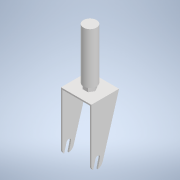
# Autodesk Inventor part: frontwheelFork
Saved by Autodesk Inventor 2022.2 (Build 262287010, 287A)
## iProperties
Created: 2022-04-06
Part Number: frontwheelFork
Material: Generic
Document SubType Name: Modeling
Designer: Finn Oriwohl
Density: 1 g/cm^3
Appearance: Default
Author: Finn Oriwohl
Autodesk Inventor part; units mm, degrees
ref_plane "YZ Plane" through (0, 0, 0) normal (1, 0, 0) x (0, 1, 0)
ref_plane "XZ Plane" through (0, 0, 0) normal (0, 1, 0) x (-1, 0, 0)
ref_plane "XY Plane" through (0, 0, 0) normal (0, 0, 1) x (1, 0, 0)
sketch "Sketch1" plane through (0, 0, 0) normal (0, 1, 0) x (-1, 0, 0)
  line L0 (32.75, 30) -> (-32.75, 30)
  line L1 (-32.75, 30) -> (-32.75, -30)
  line L2 (-32.75, -30) -> (32.75, -30)
  line L3 (32.75, -30) -> (32.75, 30)
  line L4 (32.75, 30) -> (-32.75, -30) construction
  line L5 (-32.75, 30) -> (32.75, -30) construction
  line L6 (-5.7735, -10) -> (-11.547, 0)
  line L7 (-11.547, 0) -> (-5.7735, 10)
  line L8 (-5.7735, 10) -> (5.7735, 10)
  line L9 (5.7735, 10) -> (11.547, 0)
  line L10 (11.547, 0) -> (5.7735, -10)
  line L11 (5.7735, -10) -> (-5.7735, -10)
  point P0 (0, 0)
  point P1 (0, 0)
  point P2 (0, 10)
  dimension "d1" = 65.5
  dimension "d2" = 60
  dimension "d3" = 20
  constraints: 24 end point, 2 parallel, 1 coincident, 1 horizontal, 1 midpoint, 1 perpendicular, 13 other
  measures "d1" distance of L2.end L1.end
  measures "d2" distance of L1.end L0.end
  measures "d3" distance from line of L11 point (0, 10)
extrude "Extrusion1" add sketch "Sketch1" against normal blind 3
extrude "Extrusion2" add sketch "Sketch1" along normal blind 10 and the other way blind 3 contours L6 L7 L8 L9 L10 L11
sketch "Sketch2" plane through (0, 10, 0) normal (0, 1, 0) x (1, 0, 0)
  circle A0 centre (0, 0) radius 14.25
  dimension "d10" = 28.5
  constraints: 1 centre point, 1 coincident
  measures "d10" diameter of A0
extrude "Extrusion3" add sketch "Sketch2" along normal blind 110
sketch "Sketch3" plane through (0, -3, 0) normal (0, -1, 0) x (1, 0, 0)
  line L0 (32.75, -30) -> (32.75, 30) projected
  line L1 (32.75, 30) -> (-32.75, 30) projected
  line L2 (-32.75, 30) -> (-32.75, -30) projected
  line L3 (-32.75, -30) -> (32.75, -30) projected
  line L4 (29.75, 30) -> (29.75, -30)
  line L5 (0, 0) -> (0, -7) construction
  line L6 (-29.75, 30) -> (-29.75, -30)
  dimension "d13" = 3
  constraints: 6 end point, 2 point on line, 2 symmetric about line, 1 perpendicular, 1 vertical
  measures "d13" distance between parallel lines of L0 L4
extrude "Extrusion4" add sketch "Sketch3" along normal blind 127 contours L3 L4 L1 L0 | L3 L2 L1 L6
sketch "Sketch4" plane through (32.75, 0, 30) normal (1, 0, 0) x (0, 0, -1)
  line L0 (0, 0) -> (60, 0) projected
  line L1 (0, 0) -> (0, -130) projected
  line L2 (60, -130) -> (0, -130) projected
  line L3 (60, 0) -> (60, -130) projected
  line L4 (0, 0) -> (60, 0) projected
  line L5 (60, 0) -> (21.1215, -130)
  arc A0 (18.8567, -108.1886) -> (9.1837, -105.6571) centre (14, -107) ccw
  line L6 (14, -107) -> (28, -107) construction
  line L7 (0, 0) -> (0, -130) projected
  line L8 (9.1837, -105.6571) -> (2, -131.4205)
  line L9 (2, -131.4205) -> (12.5394, -134)
  line L10 (12.5394, -134) -> (18.8567, -108.1886)
  arc A1 (0, -114.9326) -> (24.5531, -118.5255) centre (12.5394, -114.9326) ccw
  point P0 (30, 0)
  point P1 (14.163, -127.3665)
  point P2 (4.0294, -124.1422)
  point P3 (2.3961, -130)
  point P4 (13.5184, -130)
  dimension "d16" = 130
  dimension "d18" = 10
  dimension "d19" = 107
  dimension "d20" = 14
  dimension "d23" = 14
  constraints: 10 end point, 4 point on circle, 4 point on line, 4 tangent, 2 centre point, 1 horizontal
  measures "d16" distance between parallel lines of L2 L0
  measures "d18" diameter of A0
  measures "d19" distance from line of L0 L6.start
  measures "d20" distance of L6.start L6.end
  measures "d23" distance from line of L1 L6.start
extrude "Extrusion5" cut sketch "Sketch4" against normal blind 127 contours L3 L2 L5 | A1 L8 L2 L1 | L5 L2 L10 A1 | A1 L10 L2 L8 | L8 A0 L10 A1 | L2 L10 L9 L8
equation "\"d23\" = d20"
body "Solid1"
